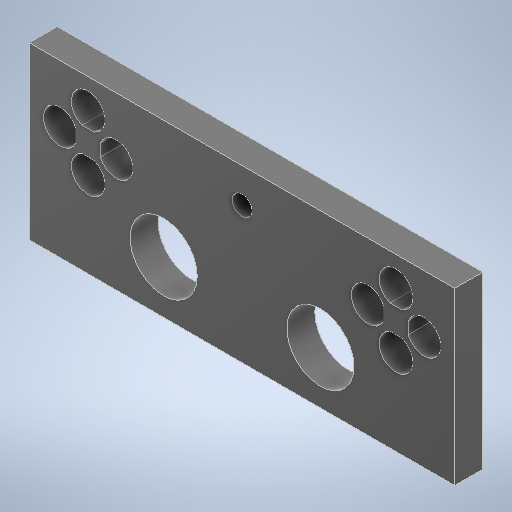
# Autodesk Inventor part: kryt_kontroleru
Saved by Autodesk Inventor 2025 (Build 290162000, 162)
## iProperties
Created: 2024-04-29
Part Number: kryt_kontroleru
Material: PC/ABS plast
Document SubType Name: Modeling
Designer: dande
Density: 1.1 g/cm^3
Appearance: Hladká – černá
Author: dande
Autodesk Inventor part; units mm, degrees
(part 1 of 2)
ref_plane "YZ Plane" through (0, 0, 0) normal (1, 0, 0) x (0, 1, 0)
ref_plane "XZ Plane" through (0, 0, 0) normal (0, 1, 0) x (-1, 0, 0)
ref_plane "XY Plane" through (0, 0, 0) normal (0, 0, 1) x (1, 0, 0)
sketch "Náčrt1" plane through (0, 0, 0) normal (0, 0, 1) x (1, 0, 0)
  line L0 (-95.6159, 0) -> (114.3841, 0) projected
  line L1 (0, 43.5277) -> (0, -40.8923) projected
  line L2 (84.3841, 31.1677) -> (-65.6159, 31.1677)
  arc A0 (-43.4618, 15.5677) -> (-47.7699, 15.5677) centre (-45.6159, 21.1677) ccw
  line L3 (-15.1159, 27.1677) -> (-15.1159, 7.1677)
  line L4 (-15.1159, 7.1677) -> (-5.1159, 7.1677)
  line L5 (-5.1159, 7.1677) -> (-15.1159, 7.1677)
  line L6 (-15.1159, 7.1677) -> (-15.1159, 27.1677)
  line L7 (-5.1159, 27.1677) -> (-15.1159, 27.1677)
  line L8 (-5.1159, 7.1677) -> (-5.1159, 27.1677)
  line L9 (-5.1159, 27.1677) -> (-5.1159, 7.1677)
  line L10 (-15.1159, 27.1677) -> (-5.1159, 27.1677)
  line L11 (-37.7159, 8.9177) -> (-37.7159, 8.4177)
  line L12 (-37.7159, 13.4177) -> (-38.5159, 13.4177)
  line L13 (-38.5159, 8.9177) -> (-37.7159, 8.9177)
  line L14 (-38.5159, 8.4177) -> (-38.5159, 8.9177)
  line L15 (-43.3659, -0.9323) -> (-43.3659, -1.7323)
  line L16 (-43.3659, -1.7323) -> (-43.3659, -0.9323)
  line L17 (-48.3659, 18.2677) -> (-48.3659, 19.0677)
  line L18 (-48.3659, 19.0677) -> (-48.3659, 18.2677)
  line L19 (-48.3659, 19.0677) -> (-47.8659, 19.0677)
  line L20 (-47.8659, 19.0677) -> (-48.3659, 19.0677)
  line L21 (-47.8659, 19.0677) -> (-47.8659, 18.2677)
  line L22 (-47.8659, 18.2677) -> (-47.8659, 19.0677)
  line L23 (-47.8659, 18.2677) -> (-48.3659, 18.2677)
  line L24 (-48.3659, 18.2677) -> (-47.8659, 18.2677)
  line L25 (-48.3659, 24.0677) -> (-48.3659, 23.2677)
  line L26 (-48.3659, 3.2677) -> (-48.3659, 4.0677)
  line L27 (-48.3659, 4.0677) -> (-48.3659, 3.2677)
  line L28 (-48.3659, -0.9323) -> (-47.8659, -0.9323)
  line L29 (-48.3659, -1.7323) -> (-47.8659, -1.7323)
  line L30 (-42.8659, -1.7323) -> (-43.3659, -1.7323)
  line L31 (-42.8659, -0.9323) -> (-43.3659, -0.9323)
  line L32 (-47.8659, 4.0677) -> (-48.3659, 4.0677)
  line L33 (-48.3659, 3.2677) -> (-47.8659, 3.2677)
  line L34 (-47.8659, -0.9323) -> (-48.3659, -0.9323)
  line L35 (-38.5159, 8.9177) -> (-38.5159, 8.4177)
  circle A1 centre (-63.1159, 28.6677) radius 0.5
  circle A2 centre (-63.1159, 28.6677) radius 0.5
  line L36 (-65.6159, 31.1677) -> (-65.6159, -28.8323)
  line L37 (-65.6159, 31.1677) -> (-65.6159, -28.8323)
  circle A3 centre (-63.1159, -26.3323) radius 0.5
  circle A4 centre (-63.1159, -26.3323) radius 0.5
  line L38 (-65.6159, -28.8323) -> (84.3841, -28.8323)
  line L39 (-65.6159, -28.8323) -> (84.3841, -28.8323)
  line L40 (84.3841, -28.8323) -> (84.3841, 31.1677)
  line L41 (84.3841, -28.8323) -> (84.3841, 31.1677)
  circle A5 centre (3.6841, 28.1677) radius 0.5
  circle A6 centre (3.6841, -18.8323) radius 0.5
  circle A7 centre (3.6841, 28.1677) radius 1.9
  circle A8 centre (3.6841, -18.8323) radius 1.9
  circle A9 centre (3.6841, 28.1677) radius 1.9
  circle A10 centre (3.6841, -18.8323) radius 1.9
  line L42 (84.3841, 31.1677) -> (-65.6159, 31.1677)
  circle A11 centre (15.0841, 28.1677) radius 0.5
  circle A12 centre (15.0841, -18.8323) radius 0.5
  circle A13 centre (15.0841, 28.1677) radius 0.5
  circle A14 centre (15.0841, -18.8323) radius 0.5
  circle A15 centre (15.0841, 28.1677) radius 1.9
  circle A16 centre (15.0841, -18.8323) radius 1.9
  circle A17 centre (15.0841, 28.1677) radius 1.9
  circle A18 centre (15.0841, -18.8323) radius 1.9
  circle A19 centre (81.8841, -26.3323) radius 0.5
  circle A20 centre (81.8841, -26.3323) radius 0.5
  circle A21 centre (81.8841, 28.6677) radius 0.5
  circle A22 centre (3.6841, 28.1677) radius 0.5
  circle A23 centre (81.8841, 28.6677) radius 0.5
  circle A24 centre (-30.6159, -0.2323) radius 0.5
  line L43 (-33.5159, 13.4177) -> (-32.7159, 13.4177)
  line L44 (-37.7159, 8.4177) -> (-37.7159, 8.9177)
  line L45 (-37.7159, 13.4177) -> (-37.7159, 13.9177)
  line L46 (-38.5159, 13.9177) -> (-37.7159, 13.9177)
  line L47 (-37.7159, 8.9177) -> (-38.5159, 8.9177)
  line L48 (-42.8659, -0.9323) -> (-42.8659, -1.7323)
  line L49 (-43.3659, -1.7323) -> (-42.8659, -1.7323)
  line L50 (-47.8659, -0.9323) -> (-47.8659, -1.7323)
  line L51 (-47.8659, -1.7323) -> (-48.3659, -1.7323)
  line L52 (-47.8659, 4.0677) -> (-47.8659, 3.2677)
  line L53 (-47.8659, 3.2677) -> (-48.3659, 3.2677)
  line L54 (-57.7159, 13.4177) -> (-57.7159, 13.9177)
  line L55 (-47.8659, -1.7323) -> (-47.8659, -0.9323)
  line L56 (-47.8659, 3.2677) -> (-47.8659, 4.0677)
  line L57 (-48.3659, 4.0677) -> (-47.8659, 4.0677)
  line L58 (-57.7159, 13.9177) -> (-57.7159, 13.4177)
  line L59 (-57.7159, 13.9177) -> (-58.5159, 13.9177)
  line L60 (-58.5159, 13.9177) -> (-57.7159, 13.9177)
  line L61 (-58.5159, 13.4177) -> (-57.7159, 13.4177)
  line L62 (-58.5159, 13.4177) -> (-58.5159, 13.9177)
  line L63 (-58.5159, 13.9177) -> (-58.5159, 13.4177)
  line L64 (-38.5159, 8.4177) -> (-37.7159, 8.4177)
  line L65 (-42.8659, -1.7323) -> (-42.8659, -0.9323)
  line L66 (-37.7159, 8.4177) -> (-38.5159, 8.4177)
  circle A25 centre (-4.1159, -0.2323) radius 0.5
  circle A26 centre (-4.1159, -0.2323) radius 0.5
  circle A27 centre (3.6841, -18.8323) radius 0.5
  circle A28 centre (-4.1159, -20.3323) radius 0.5
  circle A29 centre (-4.1159, -20.3323) radius 0.5
  line L67 (-57.7159, 13.4177) -> (-58.5159, 13.4177)
  line L68 (51.4841, 13.9177) -> (52.2841, 13.9177)
  line L69 (52.2841, 13.9177) -> (51.4841, 13.9177)
  line L70 (51.4841, 13.4177) -> (51.4841, 13.9177)
  line L71 (51.4841, 13.9177) -> (51.4841, 13.4177)
  line L72 (51.4841, 13.4177) -> (52.2841, 13.4177)
  line L73 (52.2841, 13.4177) -> (52.2841, 13.9177)
  line L74 (52.2841, 13.4177) -> (51.4841, 13.4177)
  line L75 (52.2841, 13.9177) -> (52.2841, 13.4177)
  line L76 (61.6341, 3.2677) -> (61.6341, 4.0677)
  line L77 (61.6341, 4.0677) -> (61.6341, 3.2677)
  line L78 (61.6341, 4.0677) -> (62.1341, 4.0677)
  line L79 (62.1341, 3.2677) -> (61.6341, 3.2677)
  line L80 (62.1341, 4.0677) -> (62.1341, 3.2677)
  line L81 (61.6341, 3.2677) -> (62.1341, 3.2677)
  line L82 (62.1341, 4.0677) -> (61.6341, 4.0677)
  line L83 (62.1341, 3.2677) -> (62.1341, 4.0677)
  line L84 (-42.8659, 3.2677) -> (-43.3659, 3.2677)
  line L85 (-42.8659, 4.0677) -> (-42.8659, 3.2677)
  line L86 (-42.8659, 3.2677) -> (-42.8659, 4.0677)
  line L87 (-43.3659, 4.0677) -> (-42.8659, 4.0677)
  line L88 (-42.8659, 4.0677) -> (-43.3659, 4.0677)
  line L89 (-43.3659, 3.2677) -> (-43.3659, 4.0677)
  line L90 (-43.3659, 4.0677) -> (-43.3659, 3.2677)
  line L91 (-43.3659, 3.2677) -> (-42.8659, 3.2677)
  line L92 (-58.5159, 8.4177) -> (-58.5159, 8.9177)
  line L93 (-58.5159, 8.9177) -> (-58.5159, 8.4177)
  line L94 (-57.7159, 8.9177) -> (-57.7159, 8.4177)
  line L95 (-57.7159, 8.4177) -> (-57.7159, 8.9177)
  line L96 (-57.7159, 8.4177) -> (-58.5159, 8.4177)
  line L97 (-58.5159, 8.4177) -> (-57.7159, 8.4177)
  line L98 (-58.5159, 8.9177) -> (-57.7159, 8.9177)
  line L99 (-57.7159, 8.9177) -> (-58.5159, 8.9177)
  line L100 (-47.8659, 23.2677) -> (-48.3659, 23.2677)
  line L101 (-48.3659, 23.2677) -> (-47.8659, 23.2677)
  line L102 (-48.3659, 24.0677) -> (-47.8659, 24.0677)
  line L103 (-47.8659, 24.0677) -> (-48.3659, 24.0677)
  line L104 (-48.3659, 23.2677) -> (-48.3659, 24.0677)
  line L105 (-47.8659, 24.0677) -> (-47.8659, 23.2677)
  line L106 (-47.8659, 23.2677) -> (-47.8659, 24.0677)
  line L107 (-33.5159, 8.4177) -> (-33.5159, 8.9177)
  line L108 (-33.5159, 8.9177) -> (-33.5159, 8.4177)
  line L109 (-33.5159, 8.9177) -> (-32.7159, 8.9177)
  line L110 (-32.7159, 8.9177) -> (-33.5159, 8.9177)
  line L111 (-32.7159, 8.9177) -> (-32.7159, 8.4177)
  line L112 (-32.7159, 8.4177) -> (-32.7159, 8.9177)
  line L113 (-32.7159, 8.4177) -> (-33.5159, 8.4177)
  line L114 (-33.5159, 8.4177) -> (-32.7159, 8.4177)
  line L115 (-33.5159, 13.4177) -> (-33.5159, 13.9177)
  line L116 (-33.5159, 13.9177) -> (-33.5159, 13.4177)
  line L117 (-32.7159, 13.9177) -> (-33.5159, 13.9177)
  line L118 (-32.7159, 13.4177) -> (-32.7159, 13.9177)
  line L119 (-32.7159, 13.9177) -> (-32.7159, 13.4177)
  line L120 (-33.5159, 13.9177) -> (-32.7159, 13.9177)
  circle A30 centre (-30.6159, -0.2323) radius 0.5
  circle A31 centre (-30.6159, -20.3323) radius 0.5
  circle A32 centre (-30.6159, -20.3323) radius 0.5
  line L121 (-32.7159, 13.4177) -> (-33.5159, 13.4177)
  line L122 (-37.7159, 13.9177) -> (-37.7159, 13.4177)
  line L123 (-42.8659, 18.2677) -> (-43.3659, 18.2677)
  line L124 (-43.3659, 18.2677) -> (-42.8659, 18.2677)
  line L125 (-43.3659, 18.2677) -> (-43.3659, 19.0677)
  line L126 (-43.3659, 19.0677) -> (-43.3659, 18.2677)
  line L127 (-43.3659, 19.0677) -> (-42.8659, 19.0677)
  line L128 (-42.8659, 19.0677) -> (-43.3659, 19.0677)
  line L129 (-42.8659, 19.0677) -> (-42.8659, 18.2677)
  line L130 (-42.8659, 18.2677) -> (-42.8659, 19.0677)
  line L131 (-38.5159, 13.9177) -> (-38.5159, 13.4177)
  line L132 (-37.7159, 13.9177) -> (-38.5159, 13.9177)
  line L133 (-38.5159, 13.4177) -> (-37.7159, 13.4177)
  line L134 (-38.5159, 13.4177) -> (-38.5159, 13.9177)
  line L135 (-43.3659, -0.9323) -> (-42.8659, -0.9323)
  line L136 (-48.3659, -1.7323) -> (-48.3659, -0.9323)
  line L137 (-48.3659, -0.9323) -> (-48.3659, -1.7323)
  line L138 (-53.5159, 8.9177) -> (-52.7159, 8.9177)
  line L139 (-52.7159, 8.9177) -> (-53.5159, 8.9177)
  line L140 (-52.7159, 8.9177) -> (-52.7159, 8.4177)
  line L141 (-52.7159, 8.4177) -> (-52.7159, 8.9177)
  line L142 (-52.7159, 8.4177) -> (-53.5159, 8.4177)
  line L143 (-53.5159, 8.4177) -> (-52.7159, 8.4177)
  line L144 (-53.5159, 8.4177) -> (-53.5159, 8.9177)
  line L145 (-53.5159, 8.9177) -> (-53.5159, 8.4177)
  line L146 (-53.5159, 13.9177) -> (-52.7159, 13.9177)
  line L147 (-52.7159, 13.9177) -> (-53.5159, 13.9177)
  line L148 (-52.7159, 13.9177) -> (-52.7159, 13.4177)
  line L149 (-52.7159, 13.4177) -> (-52.7159, 13.9177)
  line L150 (-52.7159, 13.4177) -> (-53.5159, 13.4177)
  line L151 (-53.5159, 13.4177) -> (-52.7159, 13.4177)
  line L152 (-53.5159, 13.4177) -> (-53.5159, 13.9177)
  line L153 (-53.5159, 13.9177) -> (-53.5159, 13.4177)
  line L154 (56.4841, 13.9177) -> (56.4841, 13.4177)
  line L155 (56.4841, 13.4177) -> (56.4841, 13.9177)
  line L156 (57.2841, 13.4177) -> (56.4841, 13.4177)
  line L157 (57.2841, 13.9177) -> (57.2841, 13.4177)
  line L158 (57.2841, 13.4177) -> (57.2841, 13.9177)
  line L159 (56.4841, 13.4177) -> (57.2841, 13.4177)
  line L160 (57.2841, 13.9177) -> (56.4841, 13.9177)
  line L161 (56.4841, 13.9177) -> (57.2841, 13.9177)
  line L162 (66.6341, 4.0677) -> (66.6341, 3.2677)
  line L163 (66.6341, 3.2677) -> (66.6341, 4.0677)
  line L164 (67.1341, 18.2677) -> (66.6341, 18.2677)
  line L165 (66.6341, 18.2677) -> (67.1341, 18.2677)
  line L166 (66.6341, 18.2677) -> (66.6341, 19.0677)
  line L167 (66.6341, 19.0677) -> (67.1341, 19.0677)
  line L168 (67.1341, 19.0677) -> (66.6341, 19.0677)
  line L169 (66.6341, 19.0677) -> (66.6341, 18.2677)
  line L170 (67.1341, 19.0677) -> (67.1341, 18.2677)
  line L171 (67.1341, 18.2677) -> (67.1341, 19.0677)
  line L172 (66.6341, 24.0677) -> (67.1341, 24.0677)
  line L173 (67.1341, 24.0677) -> (66.6341, 24.0677)
  line L174 (67.1341, 23.2677) -> (66.6341, 23.2677)
  line L175 (67.1341, 24.0677) -> (67.1341, 23.2677)
  line L176 (67.1341, 23.2677) -> (67.1341, 24.0677)
  line L177 (66.6341, 23.2677) -> (67.1341, 23.2677)
  line L178 (71.4841, 8.9177) -> (72.2841, 8.9177)
  line L179 (72.2841, 8.9177) -> (71.4841, 8.9177)
  line L180 (72.2841, 8.9177) -> (72.2841, 8.4177)
  line L181 (71.4841, 8.4177) -> (71.4841, 8.9177)
  line L182 (72.2841, 8.4177) -> (71.4841, 8.4177)
  line L183 (71.4841, 8.4177) -> (72.2841, 8.4177)
  line L184 (72.2841, 8.4177) -> (72.2841, 8.9177)
  line L185 (71.4841, 8.9177) -> (71.4841, 8.4177)
  line L186 (66.6341, 23.2677) -> (66.6341, 24.0677)
  line L187 (66.6341, 24.0677) -> (66.6341, 23.2677)
  line L188 (76.4841, 8.9177) -> (76.4841, 8.4177)
  line L189 (76.4841, 8.4177) -> (76.4841, 8.9177)
  line L190 (76.4841, 8.9177) -> (77.2841, 8.9177)
  line L191 (77.2841, 8.9177) -> (76.4841, 8.9177)
  line L192 (77.2841, 8.9177) -> (77.2841, 8.4177)
  line L193 (77.2841, 8.4177) -> (77.2841, 8.9177)
  line L194 (66.6341, 4.0677) -> (67.1341, 4.0677)
  line L195 (67.1341, 4.0677) -> (66.6341, 4.0677)
  line L196 (77.2841, 8.4177) -> (76.4841, 8.4177)
  line L197 (76.4841, 8.4177) -> (77.2841, 8.4177)
  line L198 (67.1341, 3.2677) -> (67.1341, 4.0677)
  line L199 (66.6341, 3.2677) -> (67.1341, 3.2677)
  line L200 (67.1341, 3.2677) -> (66.6341, 3.2677)
  line L201 (67.1341, 4.0677) -> (67.1341, 3.2677)
  line L202 (51.4841, 8.4177) -> (51.4841, 8.9177)
  line L203 (51.4841, 8.9177) -> (51.4841, 8.4177)
  line L204 (52.2841, 8.9177) -> (51.4841, 8.9177)
  line L205 (52.2841, 8.9177) -> (52.2841, 8.4177)
  line L206 (51.4841, 8.9177) -> (52.2841, 8.9177)
  line L207 (52.2841, 8.4177) -> (52.2841, 8.9177)
  line L208 (52.2841, 8.4177) -> (51.4841, 8.4177)
  line L209 (51.4841, 8.4177) -> (52.2841, 8.4177)
  line L210 (62.1341, -1.7323) -> (62.1341, -0.9323)
  line L211 (62.1341, -0.9323) -> (62.1341, -1.7323)
  line L212 (61.6341, -1.7323) -> (61.6341, -0.9323)
  line L213 (61.6341, -0.9323) -> (61.6341, -1.7323)
  line L214 (61.6341, -0.9323) -> (62.1341, -0.9323)
  line L215 (62.1341, -1.7323) -> (61.6341, -1.7323)
  line L216 (61.6341, -1.7323) -> (62.1341, -1.7323)
  line L217 (62.1341, 18.2677) -> (61.6341, 18.2677)
  line L218 (61.6341, 18.2677) -> (62.1341, 18.2677)
  line L219 (71.4841, 13.4177) -> (71.4841, 13.9177)
  line L220 (71.4841, 13.9177) -> (71.4841, 13.4177)
  line L221 (71.4841, 13.4177) -> (72.2841, 13.4177)
  line L222 (62.1341, -0.9323) -> (61.6341, -0.9323)
  line L223 (72.2841, 13.4177) -> (71.4841, 13.4177)
  line L224 (72.2841, 13.9177) -> (71.4841, 13.9177)
  line L225 (72.2841, 13.4177) -> (72.2841, 13.9177)
  line L226 (72.2841, 13.9177) -> (72.2841, 13.4177)
  line L227 (71.4841, 13.9177) -> (72.2841, 13.9177)
  line L228 (-43.3659, 24.0677) -> (-42.8659, 24.0677)
  line L229 (-42.8659, 24.0677) -> (-43.3659, 24.0677)
  line L230 (-42.8659, 23.2677) -> (-43.3659, 23.2677)
  line L231 (-43.3659, 23.2677) -> (-42.8659, 23.2677)
  line L232 (-42.8659, 24.0677) -> (-42.8659, 23.2677)
  line L233 (-42.8659, 23.2677) -> (-42.8659, 24.0677)
  line L234 (-43.3659, 24.0677) -> (-43.3659, 23.2677)
  line L235 (-43.3659, 23.2677) -> (-43.3659, 24.0677)
  line L236 (-36.6159, -16.6323) -> (-40.6159, -16.6323)
  line L237 (-36.6159, -16.6323) -> (-36.6159, -4.6323)
  line L238 (-36.6159, -4.6323) -> (-36.6159, -16.6323)
  line L239 (-36.6159, -4.6323) -> (-40.6159, -4.6323)
  line L240 (-40.6159, -4.6323) -> (-36.6159, -4.6323)
  line L241 (-40.6159, -4.6323) -> (-40.6159, -16.6323)
  line L242 (-40.6159, -16.6323) -> (-40.6159, -4.6323)
  line L243 (-40.6159, -16.6323) -> (-36.6159, -16.6323)
  line L244 (23.8841, 7.1677) -> (23.8841, 27.1677)
  line L245 (23.8841, 27.1677) -> (23.8841, 7.1677)
  line L246 (23.8841, 7.1677) -> (33.8841, 7.1677)
  line L247 (33.8841, 7.1677) -> (33.8841, 27.1677)
  line L248 (33.8841, 27.1677) -> (23.8841, 27.1677)
  line L249 (33.8841, 27.1677) -> (33.8841, 7.1677)
  line L250 (23.8841, 27.1677) -> (33.8841, 27.1677)
  line L251 (33.8841, 7.1677) -> (23.8841, 7.1677)
  circle A33 centre (22.8841, -0.9323) radius 0.5
  circle A34 centre (22.8841, -21.0323) radius 0.5
  circle A35 centre (22.8841, -21.0323) radius 0.5
  circle A36 centre (49.3841, -0.9323) radius 0.5
  circle A37 centre (49.3841, -0.9323) radius 0.5
  circle A38 centre (49.3841, -21.0323) radius 0.5
  circle A39 centre (49.3841, -21.0323) radius 0.5
  circle A40 centre (22.8841, -0.9323) radius 0.5
  line L252 (56.4841, 8.9177) -> (57.2841, 8.9177)
  line L253 (57.2841, 8.9177) -> (56.4841, 8.9177)
  line L254 (57.2841, 8.9177) -> (57.2841, 8.4177)
  line L255 (57.2841, 8.4177) -> (57.2841, 8.9177)
  line L256 (57.2841, 8.4177) -> (56.4841, 8.4177)
  line L257 (56.4841, 8.4177) -> (57.2841, 8.4177)
  line L258 (56.4841, 8.4177) -> (56.4841, 8.9177)
  line L259 (56.4841, 8.9177) -> (56.4841, 8.4177)
  line L260 (59.3841, -16.6323) -> (55.3841, -16.6323)
  line L261 (55.3841, -16.6323) -> (59.3841, -16.6323)
  line L262 (55.3841, -4.6323) -> (55.3841, -16.6323)
  line L263 (55.3841, -16.6323) -> (55.3841, -4.6323)
  line L264 (59.3841, -16.6323) -> (59.3841, -4.6323)
  line L265 (59.3841, -4.6323) -> (59.3841, -16.6323)
  line L266 (59.3841, -4.6323) -> (55.3841, -4.6323)
  line L267 (55.3841, -4.6323) -> (59.3841, -4.6323)
  line L268 (67.1341, -1.7323) -> (66.6341, -1.7323)
  line L269 (66.6341, -1.7323) -> (67.1341, -1.7323)
  line L270 (66.6341, -1.7323) -> (66.6341, -0.9323)
  line L271 (66.6341, -0.9323) -> (66.6341, -1.7323)
  line L272 (66.6341, -0.9323) -> (67.1341, -0.9323)
  line L273 (67.1341, -0.9323) -> (66.6341, -0.9323)
  line L274 (67.1341, -0.9323) -> (67.1341, -1.7323)
  line L275 (67.1341, -1.7323) -> (67.1341, -0.9323)
  line L276 (76.4841, 13.4177) -> (76.4841, 13.9177)
  line L277 (76.4841, 13.9177) -> (76.4841, 13.4177)
  line L278 (76.4841, 13.9177) -> (77.2841, 13.9177)
  line L279 (77.2841, 13.9177) -> (76.4841, 13.9177)
  line L280 (77.2841, 13.9177) -> (77.2841, 13.4177)
  line L281 (77.2841, 13.4177) -> (77.2841, 13.9177)
  line L282 (77.2841, 13.4177) -> (76.4841, 13.4177)
  line L283 (76.4841, 13.4177) -> (77.2841, 13.4177)
  line L284 (61.6341, 18.2677) -> (61.6341, 19.0677)
  line L285 (61.6341, 19.0677) -> (61.6341, 18.2677)
  line L286 (62.1341, 19.0677) -> (62.1341, 18.2677)
  line L287 (62.1341, 18.2677) -> (62.1341, 19.0677)
  line L288 (61.6341, 19.0677) -> (62.1341, 19.0677)
  line L289 (62.1341, 19.0677) -> (61.6341, 19.0677)
  line L290 (62.1341, 23.2677) -> (61.6341, 23.2677)
  line L291 (61.6341, 23.2677) -> (62.1341, 23.2677)
  line L292 (61.6341, 24.0677) -> (61.6341, 23.2677)
  line L293 (62.1341, 23.2677) -> (62.1341, 24.0677)
  line L294 (62.1341, 24.0677) -> (61.6341, 24.0677)
  line L295 (62.1341, 24.0677) -> (62.1341, 23.2677)
  line L296 (61.6341, 24.0677) -> (62.1341, 24.0677)
  line L297 (61.6341, 23.2677) -> (61.6341, 24.0677)
  line L298 (20.3841, -23.8323) -> (54.3841, -23.8323)
  line L299 (20.3841, -23.8323) -> (54.3841, -23.8323)
  line L300 (54.3841, -23.8323) -> (54.3841, 2.5677)
  line L301 (54.3841, -23.8323) -> (54.3841, 2.5677)
  line L302 (30.8841, -17.1323) -> (30.8841, -4.1323)
  line L303 (43.8841, -17.1323) -> (30.8841, -17.1323)
  line L304 (43.8841, -17.1323) -> (43.8841, -4.1323)
  circle A41 centre (49.3841, -21.0323) radius 0.5
  circle A42 centre (49.3841, -21.0323) radius 0.5
  line L305 (30.8841, -4.1323) -> (43.8841, -4.1323)
  line L306 (54.3841, 2.5677) -> (20.3841, 2.5677)
  line L307 (54.3841, 2.5677) -> (20.3841, 2.5677)
  circle A43 centre (22.8841, -0.9323) radius 0.5
  circle A44 centre (22.8841, -0.9323) radius 0.5
  circle A45 centre (22.8841, -21.0323) radius 0.5
  line L308 (20.3841, 2.5677) -> (20.3841, -23.8323)
  line L309 (20.3841, 2.5677) -> (20.3841, -23.8323)
  circle A46 centre (49.3841, -0.9323) radius 0.5
  circle A47 centre (49.3841, -0.9323) radius 0.5
  line L310 (53.3841, -10.8823) -> (53.3841, -10.3823)
  line L311 (43.8841, -4.1323) -> (30.8841, -4.1323)
  line L312 (43.8841, -4.1323) -> (43.8841, -17.1323)
  line L313 (53.3841, -3.8823) -> (53.3841, -4.3823)
  line L314 (53.3841, -4.3823) -> (53.3841, -3.8823)
  line L315 (53.3841, -7.6323) -> (55.3841, -7.6323)
  line L316 (53.3841, -7.6323) -> (55.3841, -7.6323)
  line L317 (55.3841, -7.1323) -> (55.3841, -7.6323)
  line L318 (55.3841, -7.6323) -> (55.3841, -7.1323)
  line L319 (53.3841, -7.1323) -> (55.3841, -7.1323)
  line L320 (53.3841, -7.1323) -> (55.3841, -7.1323)
  line L321 (53.3841, -4.3823) -> (55.3841, -4.3823)
  line L322 (55.3841, -4.3823) -> (55.3841, -3.8823)
  line L323 (53.3841, -3.8823) -> (55.3841, -3.8823)
  line L324 (55.3841, -3.8823) -> (55.3841, -4.3823)
  line L325 (53.3841, -4.3823) -> (55.3841, -4.3823)
  line L326 (53.3841, -3.8823) -> (55.3841, -3.8823)
  line L327 (53.3841, -18.1323) -> (53.3841, -3.1323)
  line L328 (53.3841, -3.1323) -> (53.3841, -18.1323)
  line L329 (53.3841, -3.1323) -> (50.3841, -3.1323)
  line L330 (50.3841, -3.1323) -> (53.3841, -3.1323)
  line L331 (50.3841, -3.1323) -> (50.3841, -18.1323)
  line L332 (50.3841, -18.1323) -> (50.3841, -3.1323)
  line L333 (50.3841, -18.1323) -> (53.3841, -18.1323)
  line L334 (53.3841, -18.1323) -> (50.3841, -18.1323)
  line L335 (53.3841, -17.3823) -> (53.3841, -16.8823)
  line L336 (53.3841, -7.6323) -> (53.3841, -7.1323)
  line L337 (53.3841, -7.1323) -> (53.3841, -7.6323)
  line L338 (53.3841, -16.8823) -> (53.3841, -17.3823)
  line L339 (53.3841, -13.6323) -> (55.3841, -13.6323)
  line L340 (55.3841, -13.6323) -> (55.3841, -14.1323)
  line L341 (53.3841, -14.1323) -> (55.3841, -14.1323)
  line L342 (53.3841, -14.1323) -> (55.3841, -14.1323)
  line L343 (55.3841, -14.1323) -> (55.3841, -13.6323)
  line L344 (53.3841, -13.6323) -> (53.3841, -14.1323)
  line L345 (53.3841, -13.6323) -> (55.3841, -13.6323)
  line L346 (53.3841, -14.1323) -> (53.3841, -13.6323)
  line L347 (53.3841, -10.3823) -> (55.3841, -10.3823)
  line L348 (53.3841, -10.3823) -> (55.3841, -10.3823)
  line L349 (53.3841, -10.8823) -> (55.3841, -10.8823)
  line L350 (53.3841, -10.3823) -> (53.3841, -10.8823)
  line L351 (53.3841, -10.8823) -> (55.3841, -10.8823)
  line L352 (55.3841, -10.8823) -> (55.3841, -10.3823)
  line L353 (55.3841, -10.3823) -> (55.3841, -10.8823)
  circle A48 centre (22.8841, -21.0323) radius 0.5
  line L354 (38.1341, -11.3823) -> (36.6341, -11.3823)
  line L355 (36.6341, -11.3823) -> (36.6341, -9.8823)
  line L356 (36.6341, -9.8823) -> (38.1341, -9.8823)
  line L357 (38.1341, -9.8823) -> (38.1341, -11.3823)
  circle A49 centre (37.3841, -10.6323) radius 3
  circle A50 centre (37.3841, -10.6323) radius 8.5
  circle A51 centre (37.3841, -10.6323) radius 8.5
  circle A52 centre (37.3841, -10.6323) radius 9.5
  circle A53 centre (37.3841, -10.6323) radius 9.5
  circle A54 centre (37.3841, -10.6323) radius 12
  circle A55 centre (37.3841, -10.6323) radius 3
  line L358 (30.8841, -4.1323) -> (30.8841, -17.1323)
  line L359 (30.8841, -17.1323) -> (43.8841, -17.1323)
  line L360 (38.1341, -11.3823) -> (36.6341, -11.3823)
  line L361 (38.1341, -9.8823) -> (38.1341, -11.3823)
  line L362 (36.6341, -9.8823) -> (38.1341, -9.8823)
  line L363 (36.6341, -11.3823) -> (36.6341, -9.8823)
  line L364 (53.3841, -16.8823) -> (55.3841, -16.8823)
  line L365 (55.3841, -16.8823) -> (55.3841, -17.3823)
  line L366 (53.3841, -17.3823) -> (55.3841, -17.3823)
  line L367 (53.3841, -17.3823) -> (55.3841, -17.3823)
  line L368 (55.3841, -17.3823) -> (55.3841, -16.8823)
  line L369 (53.3841, -16.8823) -> (55.3841, -16.8823)
  line L370 (-1.6159, 2.5677) -> (-35.6159, 2.5677)
  line L371 (-1.6159, 2.5677) -> (-35.6159, 2.5677)
  line L372 (-35.6159, 2.5677) -> (-35.6159, -23.8323)
  line L373 (-35.6159, 2.5677) -> (-35.6159, -23.8323)
  line L374 (-12.1159, -4.1323) -> (-12.1159, -17.1323)
  line L375 (-25.1159, -4.1323) -> (-12.1159, -4.1323)
  line L376 (-25.1159, -4.1323) -> (-25.1159, -17.1323)
  circle A56 centre (-30.6159, -0.2323) radius 0.5
  circle A57 centre (-30.6159, -0.2323) radius 0.5
  line L377 (-12.1159, -17.1323) -> (-25.1159, -17.1323)
  line L378 (-35.6159, -23.8323) -> (-1.6159, -23.8323)
  line L379 (-35.6159, -23.8323) -> (-1.6159, -23.8323)
  circle A58 centre (-4.1159, -20.3323) radius 0.5
  circle A59 centre (-4.1159, -20.3323) radius 0.5
  circle A60 centre (-4.1159, -0.2323) radius 0.5
  line L380 (-1.6159, -23.8323) -> (-1.6159, 2.5677)
  line L381 (-1.6159, -23.8323) -> (-1.6159, 2.5677)
  circle A61 centre (-30.6159, -20.3323) radius 0.5
  circle A62 centre (-30.6159, -20.3323) radius 0.5
  line L382 (-34.6159, -10.3823) -> (-34.6159, -10.8823)
  line L383 (-25.1159, -17.1323) -> (-12.1159, -17.1323)
  line L384 (-25.1159, -17.1323) -> (-25.1159, -4.1323)
  line L385 (-34.6159, -17.3823) -> (-34.6159, -16.8823)
  line L386 (-34.6159, -16.8823) -> (-34.6159, -17.3823)
  line L387 (-34.6159, -13.6323) -> (-36.6159, -13.6323)
  line L388 (-34.6159, -13.6323) -> (-36.6159, -13.6323)
  line L389 (-36.6159, -14.1323) -> (-36.6159, -13.6323)
  line L390 (-36.6159, -13.6323) -> (-36.6159, -14.1323)
  line L391 (-34.6159, -14.1323) -> (-36.6159, -14.1323)
  line L392 (-34.6159, -14.1323) -> (-36.6159, -14.1323)
  line L393 (-34.6159, -16.8823) -> (-36.6159, -16.8823)
  line L394 (-36.6159, -16.8823) -> (-36.6159, -17.3823)
  line L395 (-34.6159, -17.3823) -> (-36.6159, -17.3823)
  line L396 (-36.6159, -17.3823) -> (-36.6159, -16.8823)
  line L397 (-34.6159, -16.8823) -> (-36.6159, -16.8823)
  line L398 (-34.6159, -17.3823) -> (-36.6159, -17.3823)
  line L399 (-34.6159, -3.1323) -> (-34.6159, -18.1323)
  line L400 (-34.6159, -18.1323) -> (-34.6159, -3.1323)
  line L401 (-34.6159, -18.1323) -> (-31.6159, -18.1323)
  line L402 (-31.6159, -18.1323) -> (-34.6159, -18.1323)
  line L403 (-31.6159, -18.1323) -> (-31.6159, -3.1323)
  line L404 (-31.6159, -3.1323) -> (-31.6159, -18.1323)
  line L405 (-31.6159, -3.1323) -> (-34.6159, -3.1323)
  line L406 (-34.6159, -3.1323) -> (-31.6159, -3.1323)
  line L407 (-34.6159, -3.8823) -> (-34.6159, -4.3823)
  line L408 (-34.6159, -13.6323) -> (-34.6159, -14.1323)
  line L409 (-34.6159, -14.1323) -> (-34.6159, -13.6323)
  line L410 (-34.6159, -4.3823) -> (-34.6159, -3.8823)
  line L411 (-34.6159, -7.6323) -> (-36.6159, -7.6323)
  line L412 (-36.6159, -7.6323) -> (-36.6159, -7.1323)
  line L413 (-34.6159, -7.1323) -> (-36.6159, -7.1323)
  line L414 (-34.6159, -7.1323) -> (-36.6159, -7.1323)
  line L415 (-36.6159, -7.1323) -> (-36.6159, -7.6323)
  line L416 (-34.6159, -7.6323) -> (-34.6159, -7.1323)
  line L417 (-34.6159, -7.6323) -> (-36.6159, -7.6323)
  line L418 (-34.6159, -7.1323) -> (-34.6159, -7.6323)
  line L419 (-34.6159, -10.8823) -> (-36.6159, -10.8823)
  line L420 (-34.6159, -10.8823) -> (-36.6159, -10.8823)
  line L421 (-34.6159, -10.3823) -> (-36.6159, -10.3823)
  line L422 (-34.6159, -10.8823) -> (-34.6159, -10.3823)
  line L423 (-34.6159, -10.3823) -> (-36.6159, -10.3823)
  line L424 (-36.6159, -10.3823) -> (-36.6159, -10.8823)
  line L425 (-36.6159, -10.8823) -> (-36.6159, -10.3823)
  circle A63 centre (-4.1159, -0.2323) radius 0.5
  line L426 (-19.3659, -9.8823) -> (-17.8659, -9.8823)
  line L427 (-17.8659, -9.8823) -> (-17.8659, -11.3823)
  line L428 (-17.8659, -11.3823) -> (-19.3659, -11.3823)
  line L429 (-19.3659, -11.3823) -> (-19.3659, -9.8823)
  circle A64 centre (-18.6159, -10.6323) radius 3
  circle A65 centre (-18.6159, -10.6323) radius 8.5
  circle A66 centre (-18.6159, -10.6323) radius 8.5
  circle A67 centre (-18.6159, -10.6323) radius 9.5
  circle A68 centre (-18.6159, -10.6323) radius 9.5
  circle A69 centre (-18.6159, -10.6323) radius 12
  circle A70 centre (-18.6159, -10.6323) radius 3
  line L430 (-12.1159, -17.1323) -> (-12.1159, -4.1323)
  line L431 (-12.1159, -4.1323) -> (-25.1159, -4.1323)
  line L432 (-19.3659, -9.8823) -> (-17.8659, -9.8823)
  line L433 (-19.3659, -11.3823) -> (-19.3659, -9.8823)
  line L434 (-17.8659, -11.3823) -> (-19.3659, -11.3823)
  line L435 (-17.8659, -9.8823) -> (-17.8659, -11.3823)
  line L436 (-34.6159, -4.3823) -> (-36.6159, -4.3823)
  line L437 (-36.6159, -4.3823) -> (-36.6159, -3.8823)
  line L438 (-34.6159, -3.8823) -> (-36.6159, -3.8823)
  line L439 (-34.6159, -3.8823) -> (-36.6159, -3.8823)
  line L440 (-36.6159, -3.8823) -> (-36.6159, -4.3823)
  line L441 (-34.6159, -4.3823) -> (-36.6159, -4.3823)
  line L442 (13.1841, 30.1677) -> (5.5841, 30.1677)
  line L443 (5.5841, 25.1677) -> (5.5841, 30.1677)
  line L444 (5.9841, 31.4677) -> (12.7841, 31.4677)
  line L445 (12.9841, 30.8677) -> (5.7841, 30.8677)
  line L446 (13.0841, 31.4677) -> (5.6841, 31.4677)
  line L447 (5.3841, 31.4677) -> (13.3841, 31.4677)
  line L448 (5.3841, 30.8677) -> (13.3841, 30.8677)
  line L449 (13.1841, 30.8677) -> (5.5841, 30.8677)
  line L450 (13.1841, 30.8677) -> (5.5841, 30.8677)
  line L451 (5.5841, 25.1677) -> (13.1841, 25.1677)
  line L452 (13.1841, 30.1677) -> (13.1841, 30.8677)
  line L453 (13.1841, 25.1677) -> (13.1841, 30.8677)
  line L454 (13.1841, 30.1677) -> (13.1841, 25.1677)
  circle A71 centre (0.4941, 28.7977) radius 0.5
  arc A72 (-1.1159, 28.2977) -> (-1.1159, 29.2977) centre (-1.1159, 28.7977) ccw
  line L455 (-1.1159, 29.5977) -> (-1.1159, 29.2977)
  line L456 (-1.1159, 27.9977) -> (0.4941, 27.9977)
  line L457 (0.4941, 27.9977) -> (-1.1159, 27.9977)
  line L458 (-1.1159, 28.2977) -> (-1.1159, 27.9977)
  arc A73 (0.4941, 27.9977) -> (0.4941, 29.5977) centre (0.4941, 28.7977) ccw
  arc A74 (0.4941, 27.9977) -> (0.4941, 29.5977) centre (0.4941, 28.7977) ccw
  line L459 (0.4941, 29.5977) -> (-1.1159, 29.5977)
  line L460 (-1.1159, 29.5977) -> (0.4941, 29.5977)
  arc A75 (-0.6159, 30.1677) -> (-1.1159, 29.6677) centre (-0.6159, 29.6677) ccw
  circle A76 centre (3.6841, 28.1677) radius 0.5
  arc A77 (0.4941, 22.9177) -> (0.4941, 24.5177) centre (0.4941, 23.7177) ccw
  arc A78 (0.4941, 22.9177) -> (0.4941, 24.5177) centre (0.4941, 23.7177) ccw
  circle A79 centre (0.4941, 23.7177) radius 0.5
  line L461 (19.3841, 30.1677) -> (13.1841, 30.1677)
  line L462 (5.5841, 30.1677) -> (-0.6159, 30.1677)
  circle A80 centre (15.0841, 28.1677) radius 0.5
  line L463 (5.7841, 31.4677) -> (5.7841, 30.8677)
  line L464 (5.9841, 31.4677) -> (5.9841, 26.4677)
  line L465 (5.6841, 26.4677) -> (5.9841, 26.4677)
  line L466 (5.6841, 31.4677) -> (5.6841, 26.4677)
  line L467 (5.6841, 31.4677) -> (5.9841, 31.4677)
  line L468 (5.6841, 31.4677) -> (5.6841, 26.4677)
  line L469 (13.0841, 26.4677) -> (5.6841, 26.4677)
  line L470 (13.1841, 25.1677) -> (5.5841, 25.1677)
  line L471 (5.9841, 26.4677) -> (12.7841, 26.4677)
  line L472 (12.9841, 31.4677) -> (5.7841, 31.4677)
  line L473 (5.5841, 30.8677) -> (5.5841, 30.1677)
  line L474 (5.3841, 30.8677) -> (5.3841, 31.4677)
  line L475 (5.3841, 30.8677) -> (5.3841, 31.4677)
  line L476 (5.3841, 31.4677) -> (5.7841, 31.4677)
  line L477 (5.7841, 30.8677) -> (5.3841, 30.8677)
  line L478 (13.3841, 30.8677) -> (13.3841, 31.4677)
  line L479 (5.5841, 30.8677) -> (5.5841, 25.1677)
  line L480 (-1.1159, 25.7577) -> (-1.1159, 25.4577)
  line L481 (-1.1159, 25.4577) -> (0.4941, 25.4577)
  line L482 (0.4941, 25.4577) -> (-1.1159, 25.4577)
  arc A81 (0.4941, 17.8377) -> (0.4941, 19.4377) centre (0.4941, 18.6377) ccw
  arc A82 (0.4941, 17.8377) -> (0.4941, 19.4377) centre (0.4941, 18.6377) ccw
  line L483 (0.4941, 19.4377) -> (-1.1159, 19.4377)
  line L484 (-1.1159, 19.4377) -> (0.4941, 19.4377)
  circle A83 centre (0.4941, 18.6377) radius 0.5
  line L485 (-1.1159, 19.4377) -> (-1.1159, 19.1377)
  line L486 (-1.1159, 20.6777) -> (-1.1159, 20.3777)
  arc A84 (-1.1159, 18.1377) -> (-1.1159, 19.1377) centre (-1.1159, 18.6377) ccw
  line L487 (-1.1159, 17.8377) -> (0.4941, 17.8377)
  line L488 (0.4941, 17.8377) -> (-1.1159, 17.8377)
  line L489 (0.4941, 16.8977) -> (-1.1159, 16.8977)
  line L490 (-1.1159, 16.8977) -> (0.4941, 16.8977)
  arc A85 (0.4941, 15.2977) -> (0.4941, 16.8977) centre (0.4941, 16.0977) ccw
  arc A86 (0.4941, 15.2977) -> (0.4941, 16.8977) centre (0.4941, 16.0977) ccw
  circle A87 centre (0.4941, 16.0977) radius 0.5
  line L491 (-1.1159, 18.1377) -> (-1.1159, 17.8377)
  line L492 (-1.1159, 16.8977) -> (-1.1159, 16.5977)
  arc A88 (-1.1159, 15.5977) -> (-1.1159, 16.5977) centre (-1.1159, 16.0977) ccw
  line L493 (-1.1159, 15.5977) -> (-1.1159, 15.2977)
  line L494 (-1.1159, 24.5177) -> (0.4941, 24.5177)
  line L495 (0.4941, 24.5177) -> (-1.1159, 24.5177)
  line L496 (-1.1159, 24.5177) -> (-1.1159, 24.2177)
  arc A89 (-1.1159, 23.2177) -> (-1.1159, 24.2177) centre (-1.1159, 23.7177) ccw
  circle A90 centre (0.4941, 21.1777) radius 0.5
  line L497 (-1.1159, 23.2177) -> (-1.1159, 22.9177)
  line L498 (0.4941, 22.9177) -> (-1.1159, 22.9177)
  line L499 (-1.1159, 22.9177) -> (0.4941, 22.9177)
  arc A91 (0.4941, 20.3777) -> (0.4941, 21.9777) centre (0.4941, 21.1777) ccw
  arc A92 (0.4941, 20.3777) -> (0.4941, 21.9777) centre (0.4941, 21.1777) ccw
  line L500 (0.4941, 21.9777) -> (-1.1159, 21.9777)
  line L501 (-1.1159, 21.9777) -> (0.4941, 21.9777)
  line L502 (-1.1159, 21.9777) -> (-1.1159, 21.6777)
  arc A93 (-1.1159, 20.6777) -> (-1.1159, 21.6777) centre (-1.1159, 21.1777) ccw
  line L503 (-1.1159, 20.3777) -> (0.4941, 20.3777)
  line L504 (-1.1159, 15.2977) -> (0.4941, 15.2977)
  line L505 (0.4941, 15.2977) -> (-1.1159, 15.2977)
  line L506 (0.4941, 20.3777) -> (-1.1159, 20.3777)
  line L507 (-1.1159, 27.0577) -> (0.4941, 27.0577)
  line L508 (-1.1159, 27.0577) -> (-1.1159, 26.7577)
  arc A94 (-1.1159, 25.7577) -> (-1.1159, 26.7577) centre (-1.1159, 26.2577) ccw
  circle A95 centre (0.4941, 26.2577) radius 0.5
  arc A96 (0.4941, 25.4577) -> (0.4941, 27.0577) centre (0.4941, 26.2577) ccw
  arc A97 (0.4941, 25.4577) -> (0.4941, 27.0577) centre (0.4941, 26.2577) ccw
  line L509 (0.4941, 27.0577) -> (-1.1159, 27.0577)
  line L510 (-1.1159, -0.8823) -> (-1.1159, -1.1823)
  circle A98 centre (0.4941, -1.6823) radius 0.5
  line L511 (0.4941, -2.4823) -> (-1.1159, -2.4823)
  line L512 (-1.1159, 7.6777) -> (0.4941, 7.6777)
  line L513 (-1.1159, 5.1377) -> (-1.1159, 4.1977)
  arc A99 (0.4941, -2.4823) -> (0.4941, -0.8823) centre (0.4941, -1.6823) ccw
  arc A100 (0.4941, -2.4823) -> (0.4941, -0.8823) centre (0.4941, -1.6823) ccw
  line L514 (-1.1159, -2.4823) -> (0.4941, -2.4823)
  line L515 (-1.1159, -2.1823) -> (-1.1159, -2.4823)
  arc A101 (-1.1159, -2.1823) -> (-1.1159, -1.1823) centre (-1.1159, -1.6823) ccw
  arc A102 (0.4941, 7.6777) -> (0.4941, 9.2777) centre (0.4941, 8.4777) ccw
  arc A103 (0.4941, 7.6777) -> (0.4941, 9.2777) centre (0.4941, 8.4777) ccw
  line L516 (0.4941, 7.6777) -> (-1.1159, 7.6777)
  circle A104 centre (0.4941, 8.4777) radius 0.5
  line L517 (-1.1159, 7.9777) -> (-1.1159, 7.6777)
  arc A105 (-1.1159, 7.9777) -> (-1.1159, 8.9777) centre (-1.1159, 8.4777) ccw
  line L518 (-1.1159, 9.2777) -> (-1.1159, 8.9777)
  line L519 (0.4941, 9.2777) -> (-1.1159, 9.2777)
  line L520 (-1.1159, 9.2777) -> (0.4941, 9.2777)
  line L521 (-1.1159, -0.8823) -> (0.4941, -0.8823)
  line L522 (-1.1159, 5.4377) -> (-1.1159, 3.8977)
  circle A106 centre (0.4941, 3.3977) radius 0.5
  arc A107 (-1.1159, 5.4377) -> (-1.1159, 6.4377) centre (-1.1159, 5.9377) ccw
  circle A108 centre (0.4941, 8.4777) radius 0.5
  arc A109 (-1.1159, 0.3577) -> (-1.1159, 1.3577) centre (-1.1159, 0.8577) ccw
  line L523 (0.4941, -0.8823) -> (-1.1159, -0.8823)
  line L524 (19.8841, 21.9777) -> (19.8841, 22.9177)
  line L525 (19.8841, 19.1377) -> (19.8841, 20.6777)
  line L526 (19.8841, 19.4377) -> (19.8841, 20.3777)
  line L527 (19.8841, 16.8977) -> (19.8841, 17.8377)
  line L528 (19.8841, 16.5977) -> (19.8841, 18.1377)
  line L529 (19.8841, 14.3577) -> (19.8841, 15.2977)
  line L530 (19.8841, 14.0577) -> (19.8841, 15.5977)
  line L531 (19.8841, 11.8177) -> (19.8841, 12.7577)
  line L532 (19.8841, 11.5177) -> (19.8841, 13.0577)
  line L533 (19.8841, 9.2777) -> (19.8841, 10.2177)
  line L534 (19.8841, 8.9777) -> (19.8841, 10.5177)
  line L535 (19.8841, 21.6777) -> (19.8841, 23.2177)
  line L536 (-1.1159, 13.0577) -> (-1.1159, 11.5177)
  line L537 (-1.1159, 12.7577) -> (-1.1159, 11.8177)
  line L538 (-1.1159, 15.5977) -> (-1.1159, 14.0577)
  line L539 (-1.1159, 15.2977) -> (-1.1159, 14.3577)
  line L540 (-1.1159, 10.2177) -> (-1.1159, 9.2777)
  line L541 (-1.1159, 10.5177) -> (-1.1159, 8.9777)
  arc A110 (-1.1159, 7.9777) -> (-1.1159, 8.9777) centre (-1.1159, 8.4777) ccw
  arc A111 (-1.1159, 10.5177) -> (-1.1159, 11.5177) centre (-1.1159, 11.0177) ccw
  arc A112 (-1.1159, 13.0577) -> (-1.1159, 14.0577) centre (-1.1159, 13.5577) ccw
  circle A113 centre (0.4941, 16.0977) radius 0.5
  line L542 (-1.1159, 23.2177) -> (-1.1159, 21.6777)
  line L543 (-1.1159, 22.9177) -> (-1.1159, 21.9777)
  line L544 (-1.1159, 25.7577) -> (-1.1159, 24.2177)
  line L545 (-1.1159, 25.4577) -> (-1.1159, 24.5177)
  line L546 (-1.1159, 20.3777) -> (-1.1159, 19.4377)
  line L547 (-1.1159, 20.6777) -> (-1.1159, 19.1377)
  line L548 (-1.1159, 17.8377) -> (-1.1159, 16.8977)
  line L549 (-1.1159, 18.1377) -> (-1.1159, 16.5977)
  line L550 (-1.1159, 28.2977) -> (-1.1159, 26.7577)
  line L551 (-1.1159, 27.9977) -> (-1.1159, 27.0577)
  circle A114 centre (0.4941, 13.5577) radius 0.5
  circle A115 centre (0.4941, 11.0177) radius 0.5
  arc A116 (-1.1159, 15.5977) -> (-1.1159, 16.5977) centre (-1.1159, 16.0977) ccw
  circle A117 centre (0.4941, 21.1777) radius 0.5
  arc A118 (-1.1159, 25.7577) -> (-1.1159, 26.7577) centre (-1.1159, 26.2577) ccw
  arc A119 (-1.1159, 28.2977) -> (-1.1159, 29.2977) centre (-1.1159, 28.7977) ccw
  circle A120 centre (0.4941, 18.6377) radius 0.5
  circle A121 centre (15.0841, 28.1677) radius 0.5
  circle A122 centre (18.2741, 23.7177) radius 0.5
  line L552 (19.8841, 24.5177) -> (19.8841, 25.4577)
  line L553 (19.8841, 24.2177) -> (19.8841, 25.7577)
  circle A123 centre (18.2741, 26.2577) radius 0.5
  line L554 (19.8841, 27.0577) -> (19.8841, 27.9977)
  line L555 (19.8841, 26.7577) -> (19.8841, 28.2977)
  arc A124 (-1.1159, 18.1377) -> (-1.1159, 19.1377) centre (-1.1159, 18.6377) ccw
  arc A125 (-1.1159, 20.6777) -> (-1.1159, 21.6777) centre (-1.1159, 21.1777) ccw
  arc A126 (-1.1159, 23.2177) -> (-1.1159, 24.2177) centre (-1.1159, 23.7177) ccw
  circle A127 centre (3.6841, 28.1677) radius 0.5
  circle A128 centre (0.4941, 26.2577) radius 0.5
  circle A129 centre (0.4941, 28.7977) radius 0.5
  arc A130 (19.8841, 29.2977) -> (19.8841, 28.2977) centre (19.8841, 28.7977) ccw
  arc A131 (19.8841, 21.6777) -> (19.8841, 20.6777) centre (19.8841, 21.1777) ccw
  arc A132 (19.8841, 26.7577) -> (19.8841, 25.7577) centre (19.8841, 26.2577) ccw
  arc A133 (19.8841, 24.2177) -> (19.8841, 23.2177) centre (19.8841, 23.7177) ccw
  circle A134 centre (18.2741, 28.7977) radius 0.5
  circle A135 centre (0.4941, 23.7177) radius 0.5
  arc A136 (19.8841, 3.8977) -> (19.8841, 2.8977) centre (19.8841, 3.3977) ccw
  line L556 (18.2741, 2.5977) -> (19.8841, 2.5977)
  line L557 (19.8841, 2.5977) -> (18.2741, 2.5977)
  arc A137 (18.2741, 4.1977) -> (18.2741, 2.5977) centre (18.2741, 3.3977) ccw
  line L558 (18.2741, 4.1977) -> (19.8841, 4.1977)
  line L559 (19.8841, 4.1977) -> (18.2741, 4.1977)
  arc A138 (18.2741, 4.1977) -> (18.2741, 2.5977) centre (18.2741, 3.3977) ccw
  line L560 (19.8841, 6.7377) -> (18.2741, 6.7377)
  line L561 (18.2741, 6.7377) -> (19.8841, 6.7377)
  arc A139 (18.2741, 6.7377) -> (18.2741, 5.1377) centre (18.2741, 5.9377) ccw
  line L562 (18.2741, 5.1377) -> (19.8841, 5.1377)
  arc A140 (18.2741, 6.7377) -> (18.2741, 5.1377) centre (18.2741, 5.9377) ccw
  line L563 (19.8841, 6.7377) -> (19.8841, 7.6777)
  line L564 (19.8841, 6.4377) -> (19.8841, 7.9777)
  arc A141 (19.8841, 6.4377) -> (19.8841, 5.4377) centre (19.8841, 5.9377) ccw
  line L565 (19.8841, 5.1377) -> (19.8841, 5.4377)
  arc A142 (19.8841, 6.4377) -> (19.8841, 5.4377) centre (19.8841, 5.9377) ccw
  line L566 (19.8841, 6.4377) -> (19.8841, 6.7377)
  line L567 (18.2741, 10.2177) -> (19.8841, 10.2177)
  line L568 (19.8841, 10.2177) -> (18.2741, 10.2177)
  arc A143 (18.2741, 11.8177) -> (18.2741, 10.2177) centre (18.2741, 11.0177) ccw
  arc A144 (18.2741, 11.8177) -> (18.2741, 10.2177) centre (18.2741, 11.0177) ccw
  line L569 (19.8841, 10.2177) -> (19.8841, 10.5177)
  line L570 (19.8841, 11.5177) -> (19.8841, 11.8177)
  line L571 (19.8841, 11.8177) -> (18.2741, 11.8177)
  line L572 (18.2741, 11.8177) -> (19.8841, 11.8177)
  arc A145 (19.8841, 8.9777) -> (19.8841, 7.9777) centre (19.8841, 8.4777) ccw
  circle A146 centre (18.2741, 8.4777) radius 0.5
  circle A147 centre (18.2741, 11.0177) radius 0.5
  line L573 (19.8841, 12.7577) -> (19.8841, 13.0577)
  circle A148 centre (18.2741, 8.4777) radius 0.5
  arc A149 (19.8841, 8.9777) -> (19.8841, 7.9777) centre (19.8841, 8.4777) ccw
  line L574 (19.8841, 8.9777) -> (19.8841, 9.2777)
  line L575 (19.8841, 9.2777) -> (18.2741, 9.2777)
  line L576 (18.2741, 9.2777) -> (19.8841, 9.2777)
  arc A150 (18.2741, 9.2777) -> (18.2741, 7.6777) centre (18.2741, 8.4777) ccw
  arc A151 (18.2741, 9.2777) -> (18.2741, 7.6777) centre (18.2741, 8.4777) ccw
  circle A152 centre (18.2741, 13.5577) radius 0.5
  line L577 (19.8841, 14.3577) -> (18.2741, 14.3577)
  line L578 (18.2741, 14.3577) -> (19.8841, 14.3577)
  arc A153 (19.8841, 14.0577) -> (19.8841, 13.0577) centre (19.8841, 13.5577) ccw
  circle A154 centre (18.2741, 13.5577) radius 0.5
  circle A155 centre (18.2741, 16.0977) radius 0.5
  arc A156 (19.8841, 14.0577) -> (19.8841, 13.0577) centre (19.8841, 13.5577) ccw
  line L579 (19.8841, 14.0577) -> (19.8841, 14.3577)
  line L580 (19.8841, 17.8377) -> (19.8841, 18.1377)
  line L581 (18.2741, 17.8377) -> (19.8841, 17.8377)
  line L582 (19.8841, 17.8377) -> (18.2741, 17.8377)
  arc A157 (18.2741, 14.3577) -> (18.2741, 12.7577) centre (18.2741, 13.5577) ccw
  arc A158 (18.2741, 14.3577) -> (18.2741, 12.7577) centre (18.2741, 13.5577) ccw
  arc A159 (18.2741, 19.4377) -> (18.2741, 17.8377) centre (18.2741, 18.6377) ccw
  arc A160 (18.2741, 19.4377) -> (18.2741, 17.8377) centre (18.2741, 18.6377) ccw
  circle A161 centre (18.2741, 18.6377) radius 0.5
  line L583 (19.8841, 19.4377) -> (18.2741, 19.4377)
  line L584 (18.2741, 19.4377) -> (19.8841, 19.4377)
  line L585 (18.2741, 12.7577) -> (19.8841, 12.7577)
  line L586 (19.8841, 12.7577) -> (18.2741, 12.7577)
  arc A162 (19.8841, 19.1377) -> (19.8841, 18.1377) centre (19.8841, 18.6377) ccw
  circle A163 centre (18.2741, 18.6377) radius 0.5
  arc A164 (19.8841, 11.5177) -> (19.8841, 10.5177) centre (19.8841, 11.0177) ccw
  circle A165 centre (18.2741, 21.1777) radius 0.5
  arc A166 (19.8841, 16.5977) -> (19.8841, 15.5977) centre (19.8841, 16.0977) ccw
  line L587 (19.8841, 4.1977) -> (19.8841, 5.1377)
  line L588 (19.8841, 3.8977) -> (19.8841, 5.4377)
  circle A167 centre (18.2741, 3.3977) radius 0.5
  arc A168 (19.8841, 3.8977) -> (19.8841, 2.8977) centre (19.8841, 3.3977) ccw
  line L589 (19.8841, 2.5977) -> (19.8841, 2.8977)
  circle A169 centre (18.2741, 3.3977) radius 0.5
  line L590 (19.8841, 3.8977) -> (19.8841, 4.1977)
  line L591 (19.8841, 5.1377) -> (18.2741, 5.1377)
  line L592 (7.6441, -20.8323) -> (8.5841, -20.8323)
  arc A170 (-1.1159, -20.3323) -> (-0.6159, -20.8323) centre (-0.6159, -20.3323) ccw
  line L593 (19.8841, -13.5823) -> (19.8841, -12.6423)
  line L594 (-1.1159, -12.3423) -> (-1.1159, -13.8823)
  line L595 (19.8841, -13.8823) -> (19.8841, -12.3423)
  line L596 (19.8841, -16.1223) -> (19.8841, -15.1823)
  line L597 (19.8841, -16.4223) -> (19.8841, -14.8823)
  line L598 (19.8841, -18.6623) -> (19.8841, -17.7223)
  line L599 (19.8841, -18.9623) -> (19.8841, -17.4223)
  circle A171 centre (15.0841, -18.8323) radius 0.5
  circle A172 centre (15.0841, -18.8323) radius 0.5
  line L600 (19.8841, -20.3323) -> (19.8841, -20.2623)
  line L601 (19.8841, -20.3323) -> (19.8841, -19.9623)
  arc A173 (19.3841, -20.8323) -> (19.8841, -20.3323) centre (19.3841, -20.3323) ccw
  arc A174 (19.3841, -20.8323) -> (19.8841, -20.3323) centre (19.3841, -20.3323) ccw
  line L602 (12.4241, -20.8323) -> (19.3841, -20.8323)
  line L603 (12.7241, -20.8323) -> (19.3841, -20.8323)
  circle A175 centre (3.6841, -18.8323) radius 0.5
  line L604 (10.1841, -20.8323) -> (11.1241, -20.8323)
  line L605 (7.3441, -20.8323) -> (8.8841, -20.8323)
  arc A176 (-1.1159, -20.3323) -> (-0.6159, -20.8323) centre (-0.6159, -20.3323) ccw
  line L606 (-0.6159, -20.8323) -> (6.0441, -20.8323)
  line L607 (-0.6159, -20.8323) -> (6.3441, -20.8323)
  circle A177 centre (3.6841, -18.8323) radius 0.5
  line L608 (-1.1159, -12.6423) -> (-1.1159, -13.5823)
  arc A178 (19.8841, 29.6677) -> (19.3841, 30.1677) centre (19.3841, 29.6677) ccw
  line L609 (-1.1159, 2.8977) -> (-1.1159, 1.3577)
  line L610 (-1.1159, 7.6777) -> (-1.1159, 6.7377)
  line L611 (-1.1159, 7.9777) -> (-1.1159, 6.4377)
  arc A179 (19.8841, 29.6677) -> (19.3841, 30.1677) centre (19.3841, 29.6677) ccw
  line L612 (19.3841, 30.1677) -> (-0.6159, 30.1677)
  arc A180 (-0.6159, 30.1677) -> (-1.1159, 29.6677) centre (-0.6159, 29.6677) ccw
  line L613 (-1.1159, 2.5977) -> (-1.1159, 1.6577)
  line L614 (9.8841, -20.8323) -> (11.4241, -20.8323)
  line L615 (-1.1159, -7.2623) -> (-1.1159, -8.8023)
  line L616 (-1.1159, -7.5623) -> (-1.1159, -8.5023)
  line L617 (-1.1159, -4.7223) -> (-1.1159, -6.2623)
  circle A181 centre (0.4941, -11.8423) radius 0.5
  line L618 (-1.1159, -9.8023) -> (-1.1159, -11.3423)
  line L619 (-1.1159, -10.1023) -> (-1.1159, -11.0423)
  circle A182 centre (0.4941, -9.3023) radius 0.5
  circle A183 centre (0.4941, -6.7623) radius 0.5
  line L620 (-1.1159, -5.0223) -> (-1.1159, -5.9623)
  arc A184 (-1.1159, -4.7223) -> (-1.1159, -3.7223) centre (-1.1159, -4.2223) ccw
  line L621 (-1.1159, -2.4823) -> (-1.1159, -3.4223)
  line L622 (-1.1159, -2.1823) -> (-1.1159, -3.7223)
  line L623 (-1.1159, 0.0577) -> (-1.1159, -0.8823)
  line L624 (-1.1159, 0.3577) -> (-1.1159, -1.1823)
  arc A185 (-1.1159, -2.1823) -> (-1.1159, -1.1823) centre (-1.1159, -1.6823) ccw
  arc A186 (-1.1159, -7.2623) -> (-1.1159, -6.2623) centre (-1.1159, -6.7623) ccw
  arc A187 (-1.1159, -12.3423) -> (-1.1159, -11.3423) centre (-1.1159, -11.8423) ccw
  arc A188 (-1.1159, 2.8977) -> (-1.1159, 3.8977) centre (-1.1159, 3.3977) ccw
  circle A189 centre (18.2741, -1.6823) radius 0.5
  line L625 (19.8841, 1.6577) -> (19.8841, 2.5977)
  line L626 (19.8841, 1.3577) -> (19.8841, 2.8977)
  line L627 (19.8841, 7.6777) -> (19.8841, 7.9777)
  line L628 (18.2741, 7.6777) -> (19.8841, 7.6777)
  line L629 (19.8841, 7.6777) -> (18.2741, 7.6777)
  line L630 (19.8841, -0.8823) -> (19.8841, 0.0577)
  arc A190 (18.2741, -0.8823) -> (18.2741, -2.4823) centre (18.2741, -1.6823) ccw
  arc A191 (18.2741, -0.8823) -> (18.2741, -2.4823) centre (18.2741, -1.6823) ccw
  line L631 (18.2741, -0.8823) -> (19.8841, -0.8823)
  line L632 (19.8841, -0.8823) -> (18.2741, -0.8823)
  line L633 (19.8841, -1.1823) -> (19.8841, -0.8823)
  arc A192 (19.8841, -1.1823) -> (19.8841, -2.1823) centre (19.8841, -1.6823) ccw
  line L634 (19.8841, -2.4823) -> (18.2741, -2.4823)
  line L635 (18.2741, -2.4823) -> (19.8841, -2.4823)
  line L636 (19.8841, -2.4823) -> (19.8841, -2.1823)
  circle A193 centre (18.2741, 5.9377) radius 0.5
  circle A194 centre (0.4941, -14.3823) radius 0.5
  arc A195 (-1.1159, -9.8023) -> (-1.1159, -8.8023) centre (-1.1159, -9.3023) ccw
  arc A196 (-1.1159, -14.8823) -> (-1.1159, -13.8823) centre (-1.1159, -14.3823) ccw
  circle A197 centre (18.2741, 11.0177) radius 0.5
  arc A198 (19.8841, 11.5177) -> (19.8841, 10.5177) centre (19.8841, 11.0177) ccw
  arc A199 (18.2741, 1.6577) -> (18.2741, 0.0577) centre (18.2741, 0.8577) ccw
  arc A200 (18.2741, 1.6577) -> (18.2741, 0.0577) centre (18.2741, 0.8577) ccw
  line L637 (18.2741, 1.6577) -> (19.8841, 1.6577)
  line L638 (18.2741, 0.0577) -> (19.8841, 0.0577)
  line L639 (19.8841, 0.0577) -> (18.2741, 0.0577)
  line L640 (19.8841, -3.4223) -> (19.8841, -2.4823)
  line L641 (19.8841, -3.7223) -> (19.8841, -2.1823)
  line L642 (19.8841, -1.1823) -> (19.8841, 0.3577)
  arc A201 (19.8841, -1.1823) -> (19.8841, -2.1823) centre (19.8841, -1.6823) ccw
  circle A202 centre (0.4941, -1.6823) radius 0.5
  circle A203 centre (0.4941, 5.9377) radius 0.5
  circle A204 centre (18.2741, 5.9377) radius 0.5
  circle A205 centre (0.4941, -4.2223) radius 0.5
  arc A206 (19.8841, 1.3577) -> (19.8841, 0.3577) centre (19.8841, 0.8577) ccw
  arc A207 (19.8841, -3.7223) -> (19.8841, -4.7223) centre (19.8841, -4.2223) ccw
  circle A208 centre (0.4941, 0.8577) radius 0.5
  line L643 (19.8841, -8.5023) -> (19.8841, -7.5623)
  line L644 (19.8841, -5.9623) -> (19.8841, -5.0223)
  arc A209 (18.2741, -8.5023) -> (18.2741, -10.1023) centre (18.2741, -9.3023) ccw
  arc A210 (18.2741, -8.5023) -> (18.2741, -10.1023) centre (18.2741, -9.3023) ccw
  circle A211 centre (18.2741, -9.3023) radius 0.5
  line L645 (19.8841, -10.1023) -> (18.2741, -10.1023)
  line L646 (18.2741, -10.1023) -> (19.8841, -10.1023)
  line L647 (19.8841, -10.1023) -> (19.8841, -9.8023)
  arc A212 (19.8841, -8.8023) -> (19.8841, -9.8023) centre (19.8841, -9.3023) ccw
  line L648 (19.8841, -8.5023) -> (18.2741, -8.5023)
  line L649 (18.2741, -8.5023) -> (19.8841, -8.5023)
  line L650 (19.8841, -8.8023) -> (19.8841, -8.5023)
  circle A213 centre (18.2741, 0.8577) radius 0.5
  line L651 (19.8841, 0.0577) -> (19.8841, 0.3577)
  arc A214 (19.8841, 1.3577) -> (19.8841, 0.3577) centre (19.8841, 0.8577) ccw
  line L652 (19.8841, 1.6577) -> (18.2741, 1.6577)
  line L653 (19.8841, 1.3577) -> (19.8841, 1.6577)
  line L654 (19.8841, -8.8023) -> (19.8841, -7.2623)
  line L655 (19.8841, -11.3423) -> (19.8841, -9.8023)
  line L656 (19.8841, -11.0423) -> (19.8841, -10.1023)
  line L657 (19.8841, -6.2623) -> (19.8841, -4.7223)
  arc A215 (19.8841, -11.3423) -> (19.8841, -12.3423) centre (19.8841, -11.8423) ccw
  circle A216 centre (18.2741, -9.3023) radius 0.5
  arc A217 (19.8841, -6.2623) -> (19.8841, -7.2623) centre (19.8841, -6.7623) ccw
  circle A218 centre (18.2741, -4.2223) radius 0.5
  circle A219 centre (18.2741, -1.6823) radius 0.5
  circle A220 centre (18.2741, 0.8577) radius 0.5
  line L658 (19.8841, 29.5977) -> (19.8841, 29.6677)
  line L659 (19.8841, 29.2977) -> (19.8841, 29.6677)
  line L660 (-1.1159, 29.6677) -> (-1.1159, 29.2977)
  line L661 (-1.1159, 29.6677) -> (-1.1159, 29.5977)
  circle A221 centre (18.2741, -6.7623) radius 0.5
  line L662 (18.2741, -5.9623) -> (19.8841, -5.9623)
  line L663 (19.8841, -5.9623) -> (18.2741, -5.9623)